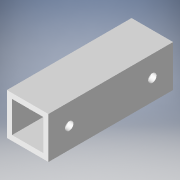
# Autodesk Inventor part: 1512898-16-A-0901
Saved by Autodesk Inventor 2017 (Build 210142000, 142)
## iProperties
Created: 2016-11-06
Part Number: 1512898-16-A-0901
Material: Generic
Document SubType Name: Modeling
Designer: gus
Mass: 21.0155 g
Surface Area: 141.431 cm^2
Volume: 21.0155 cm^3
Density: 1 g/cm^3
Appearance: Default
Author: gus
Autodesk Inventor part; units mm, degrees
ref_plane "YZ Plane" through (0, 0, 0) normal (1, 0, 0) x (0, 1, 0)
ref_plane "XZ Plane" through (0, 0, 0) normal (0, 1, 0) x (-1, 0, 0)
ref_plane "XY Plane" through (0, 0, 0) normal (0, 0, 1) x (1, 0, 0)
sketch "Sketch1" plane through (0, 0, 0) normal (0, 0, 1) x (1, 0, 0)
  line L0 (0, 0) -> (25.4, 0)
  line L1 (25.4, 0) -> (25.4, 25.4)
  line L2 (25.4, 25.4) -> (0, 25.4)
  line L3 (0, 25.4) -> (0, 0)
  line L4 (3.175, 22.225) -> (22.225, 22.225)
  line L5 (22.225, 22.225) -> (22.225, 3.175)
  line L6 (22.225, 3.175) -> (3.175, 3.175)
  line L7 (3.175, 3.175) -> (3.175, 22.225)
  dimension "d0" = 25.4
  dimension "d1" = 25.4
  dimension "d2" = 3.175
  constraints: 16 end point, 4 parallel, 2 perpendicular, 1 horizontal, 3 other
  measures "d0" distance of L2.end L1.end
  measures "d1" distance of L1.end L0.end
  measures "d2" distance between parallel lines of L2 L4
extrude "Extrusion1" add sketch "Sketch1" along normal blind 76.2
sketch "Sketch2" plane through (25.4, 0, 0) normal (1, 0, 0) x (0, 0, -1)
  line L0 (0, 0) -> (0, 25.4) projected
  line L1 (-76.2, 0) -> (-76.2, 25.4) projected
  line L2 (0, 25.4) -> (-76.2, 25.4) projected
  point P0 (-63.5, 12.7)
  point P1 (-12.7, 12.7)
  dimension "d5" = 12.7
  dimension "d6" = 12.7
  dimension "d7" = 12.7
  dimension "d8" = 12.7
  measures "d5" distance from line of L0 point (-12.7, 12.7)
  measures "d6" distance from line of L1 point (-63.5, 12.7)
  measures "d7" distance from line of L2 point (-63.5, 12.7)
  measures "d8" distance from line of L2 point (-12.7, 12.7)
hole "Hole1" at (25.4, 12.7, 63.5) at (25.4, 12.7, 12.7) direction (-1, 0, 0) diameter 5.1594 end through all
sketch "Sketch3" plane through (0, 25.4, 0) normal (0, 1, 0) x (1, 0, 0)
  line L0 (25.4, -76.2) -> (0, -76.2) projected
  line L1 (25.4, 0) -> (25.4, -76.2) projected
  point P0 (0, 0)
  point P1 (14.2875, -47.625)
  dimension "d16" = 28.575
  dimension "d17" = 11.1125
  measures "d16" distance from line of L0 point (14.287, -47.625)
  measures "d17" distance from line of L1 point (14.287, -47.625)
hole "Hole2" at (14.2875, 25.4, 47.625) direction (0, -1, 0) diameter 6.7469 end through all
body "Solid1"
